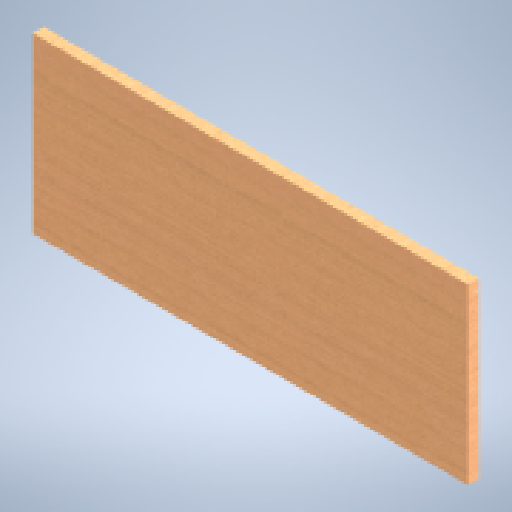
# Autodesk Inventor part: Oberseite_Shotclock
Saved by Autodesk Inventor 2024 (Build 280153000, 153)
## iProperties
Created: 2024-03-12
Part Number: Oberseite_Shotclock
Material: Holz (Kirsche)
Document SubType Name: Modeling
Designer: haniv
Density: 0.63 g/cm^3
Appearance: Kirsche - natur - schwacher Glanz
Author: haniv
Autodesk Inventor part; units mm, degrees
ref_plane "YZ Plane" through (0, 0, 0) normal (1, 0, 0) x (0, 1, 0)
ref_plane "XZ Plane" through (0, 0, 0) normal (0, 1, 0) x (-1, 0, 0)
ref_plane "XY Plane" through (0, 0, 0) normal (0, 0, 1) x (1, 0, 0)
sketch "Skizze1" plane through (0, 0, 0) normal (0, 1, 0) x (-1, 0, 0)
  line L0 (238, 95) -> (-238, 95)
  line L1 (-238, 95) -> (-238, -95)
  line L2 (-238, -95) -> (238, -95)
  line L3 (238, -95) -> (238, 95)
  point P0 (0, 0)
  point P1 (0, 95)
  point P2 (-238, 0)
  dimension "d0" = 476
  dimension "d1" = 190
  constraints: 8 end point, 2 midpoint, 2 parallel, 1 horizontal, 1 horizontal alignment, 1 perpendicular, 1 vertical alignment
  measures "d0" distance of L2.end L1.end
  measures "d1" distance of L1.end L0.end
extrude "Extrusion1" add sketch "Skizze1" along normal blind 12
sketch "Skizze2" plane through (0, 12, 0) normal (0, 1, 0) x (1, 0, 0)
  line L0 (238, -95) -> (238, 95) projected
  line L1 (238, 95) -> (-238, 95) projected
  line L2 (-238, 95) -> (-238, -95) projected
  line L3 (-238, -95) -> (238, -95) projected
  line L4 (238, -95) -> (238, 95) projected
  line L5 (238, -85) -> (-238, -85)
  line L6 (-238, -85) -> (-238, -82.8)
  line L7 (-238, -82.8) -> (238, -82.8)
  line L8 (238, -82.8) -> (238, -85)
  point P0 (0, 0)
  dimension "d4" = 10
  dimension "d5" = 2.2
  constraints: 8 end point, 2 parallel, 2 point on line, 1 horizontal, 1 perpendicular
  measures "d4" distance between parallel lines of L3 L5
  measures "d5" distance between parallel lines of L7 L5
extrude "Extrusion2" cut sketch "Skizze2" against normal blind 5 contours L5 L2 L7 L0
